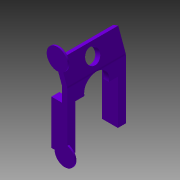
# Autodesk Inventor part: EncoderBracket
Saved by Autodesk Inventor 2014 SP1 (Build 180222100, 222)
## iProperties
Created: 2014-07-02
Part Number: EncoderBracket
Material: Generic
Document SubType Name: Modeling
Designer: Erin
Density: 1 g/cm^3
Appearance: Default
Author: Erin
Autodesk Inventor part; units mm, degrees
ref_plane "YZ Plane" through (0, 0, 0) normal (1, 0, 0) x (0, 1, 0)
ref_plane "XZ Plane" through (0, 0, 0) normal (0, 1, 0) x (-1, 0, 0)
ref_plane "XY Plane" through (0, 0, 0) normal (0, 0, 1) x (1, 0, 0)
sketch "Sketch1" plane through (0, 0, 0) normal (0, 1, 0) x (-1, 0, 0)
  line L0 (0, 0) -> (2, 0)
  line L1 (2, 0) -> (2, 22.2)
  line L2 (2, 22.2) -> (0, 22.2)
  line L3 (0, 22.2) -> (0, 0)
  line L4 (0.1206, 22.884) -> (2, 22.2)
  line L5 (2, 22.2) -> (4.7362, 29.7175)
  line L6 (4.7362, 29.7175) -> (2.8568, 30.4016)
  line L7 (2.8568, 30.4016) -> (0.1206, 22.884)
  line L8 (2, 22.2) -> (-13.9637, 28.0103) construction
  line L9 (3.7965, 30.0596) -> (1.0603, 22.542) construction
  arc A0 (2.684, 24.0794) -> (2, 20.2) centre (2, 22.2) ccw
  arc A1 (2, 20.2) -> (2.684, 24.0794) centre (2, 22.2) ccw
  circle A2 centre (3.7965, 30.0596) radius 3.9783
  circle A3 centre (1, 0) radius 3.8044
  dimension "d0" = 2
  dimension "d1" = 22.2
  dimension "d26" = 2
  dimension "d27" = 20
  dimension "d28" = 8
  constraints: 20 end point, 5 parallel, 5 point on circle, 4 centre point, 3 midpoint, 3 point on line, 2 coincident, 2 perpendicular, 1 collinear, 1 horizontal
  measures "d0" distance of L0.start L0.end
  measures "d1" distance of L0.end L1.end
  measures "d26" distance of L4.start L4.end
  measures "d27" angle of L2 L8
  measures "d28" distance of L9.start L9.end
extrude "Extrusion6" add sketch "Sketch1" along normal blind 22 contours L3 A3 L1 L0 | L3 A0 L1 A3 | A0 L4 L2 | L2 L1 A0 | L1 L5 A1 | L4 A0 L5 | L7 A2 L5 A0 | L7 L6 L5 A2 picked at (1.1123, 1.2632) picked at (3.2392, 28.8563)
extrude "Extrusion7" cut sketch "Sketch1" along normal blind 22 contours L1 L5 A1
sketch "Sketch4" plane through (-4.7362, 0, 29.7175) normal (-0.9397, 0, -0.342) x (-0.342, 0, 0.9397)
  line L0 (-8, 22) -> (0, 22) projected
  line L1 (-8, 0) -> (-8, 22) projected
  circle A0 centre (-4, 11) radius 2.7
  point P0 (-29.5452, 0)
  point P1 (-8, 11)
  point P2 (-4, 22)
  dimension "d33" = 5.4
  constraints: 2 midpoint, 1 centre point, 1 horizontal alignment, 1 vertical alignment
  measures "d33" diameter of A0
extrude "Extrusion8" cut sketch "Sketch4" against normal blind 3
sketch "Sketch5" plane through (-2, 0, 0) normal (-1, 0, 0) x (0, 0, 1)
  line L0 (0, 22) -> (22.2, 22) projected
  line L1 (0, 0) -> (0, 22) projected
  line L2 (0, 0) -> (22.2, 0) projected
  line L3 (22.2, 0) -> (22.2, 22) projected
  circle A0 centre (17.7, 11) radius 4.7
  line L4 (16.7, 22) -> (16.7, 0) construction
  line L5 (0, 19) -> (16.7, 19)
  line L6 (16.7, 19) -> (16.7, 3)
  line L7 (16.7, 3) -> (0, 3)
  line L8 (0, 3) -> (0, 19)
  line L9 (0, 22) -> (16.7, 22)
  line L10 (16.7, 22) -> (16.7, 19)
  line L11 (16.7, 19) -> (0, 19)
  line L12 (0, 19) -> (0, 22)
  line L13 (0, 3) -> (16.7, 3)
  line L14 (16.7, 3) -> (16.7, 0)
  line L15 (16.7, 0) -> (0, 0)
  line L16 (0, 0) -> (0, 3)
  point P0 (22.2, 11)
  point P1 (16.7, 11)
  point P2 (0, 11)
  dimension "d36" = 9.4
  dimension "d37" = 4.5
  dimension "d38" = 16.7
  dimension "d39" = 16
  constraints: 26 end point, 6 parallel, 4 perpendicular, 4 point on line, 3 horizontal, 3 midpoint, 2 horizontal alignment, 1 centre point
  measures "d36" diameter of A0
  measures "d37" distance from line of A0.centre L3
  measures "d38" distance between parallel lines of L4 L1
  measures "d39" distance of L5.end L6.end
extrude "Extrusion9" cut sketch "Sketch5" against normal blind 3 contours L5 L6 A0 L7 L1 | A0 L3 | L3 A0 L6 | L6 A0
extrude "Extrusion11" add sketch "Sketch1" along normal blind 0.6 contours L3 A3 L1 L0 | L0 L1 A3 L3 | A2 L5 L6 L7 | L7 L6 L5 A2
extrude "Extrusion12" add sketch "Sketch5" along normal blind 4 contours L0 L10 L5 L1 | L7 L14 L2 L1
equation "\"sp\" = 0.4"
body "Solid2"
